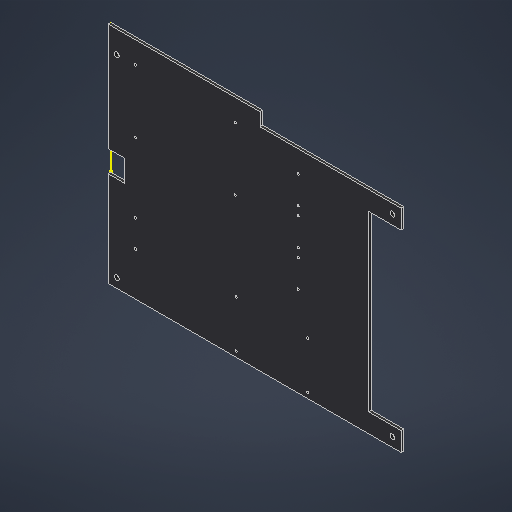
# Autodesk Inventor part: Plate-1
Saved by Autodesk Inventor 2026.2 (Build 302298010, 298A)
## iProperties
Created: 2022-04-19
Part Number: Plate-1
Material: Generic
Document SubType Name: Modeling
Designer: pollak
Density: 1 g/cm^3
Appearance: Default
Author: pollak
Autodesk Inventor part; units mm, degrees
ref_plane "YZ Plane" through (0, 0, 0) normal (1, 0, 0) x (0, 1, 0)
ref_plane "XZ Plane" through (0, 0, 0) normal (0, 1, 0) x (-1, 0, 0)
ref_plane "XY Plane" through (0, 0, 0) normal (0, 0, 1) x (1, 0, 0)
sketch "Sketch1" plane through (0, 0, 0) normal (0, 1, 0) x (-1, 0, 0)
  line L0 (135, 97.5) -> (-135, 97.5)
  line L1 (-135, 97.5) -> (-135, -97.5)
  line L2 (-135, -97.5) -> (135, -97.5)
  line L3 (135, -97.5) -> (135, 97.5)
  line L4 (135, 97.5) -> (-135, -97.5) construction
  line L5 (-135, 97.5) -> (135, -97.5) construction
  line L6 (135, 97.5) -> (-5, 97.5)
  line L7 (-5, 97.5) -> (-5, 109.5)
  line L8 (-5, 109.5) -> (135, 109.5)
  line L9 (135, 109.5) -> (135, 97.5)
  point P0 (0, 0)
  dimension "d0" = 270
  dimension "d1" = 195
  dimension "d2" = 140
  dimension "d3" = 12
  dimension "d4" = 0
  dimension "d5" = 0
  constraints: 20 end point, 4 parallel, 2 horizontal, 2 midpoint, 2 perpendicular
  measures "d0" distance of L2.end L1.end
  measures "d1" distance of L1.end L0.end
  measures "d2" distance of L7.end L8.end
  measures "d3" distance of L6.end L7.end
  measures "d4" distance between parallel lines of L3 L9
  measures "d5" distance between parallel lines of L0 L6
extrude "Extrusion1" add sketch "Sketch1" along normal blind 2.5
sketch "Mounting Holes" plane through (0, 2.5, 0) normal (0, 1, 0) x (1, 0, 0)
  line L0 (-127, -88.9) -> (127, -88.9) construction
  line L1 (127, -88.9) -> (127, 88.9) construction
  line L2 (127, 88.9) -> (-127, 88.9) construction
  line L3 (-127, 88.9) -> (-127, -88.9) construction
  line L4 (-127, -88.9) -> (127, 88.9) construction
  line L5 (127, -88.9) -> (-127, 88.9) construction
  point P0 (0, 0)
  dimension "d32" = 254
  dimension "d33" = 177.8
  constraints: 12 end point, 4 coincident, 2 midpoint, 2 parallel, 1 horizontal, 1 perpendicular
  measures "d32" distance of L2.end L1.end
  measures "d33" distance of L1.end L0.end
hole "Hole3" at (-127, 2.5, -88.9) at (127, 2.5, -88.9) at (127, 2.5, 88.9) at (-127, 2.5, 88.9) direction (0, -1, 0) diameter 4.5 end through all
sketch "Cut" plane through (0, 2.5, 0) normal (0, 1, 0) x (1, 0, 0)
  line L0 (135, 80) -> (105, 80)
  line L1 (105, 80) -> (105, -80)
  line L2 (105, -80) -> (135, -80)
  line L3 (135, -80) -> (135, 80)
  line L4 (135, 80) -> (105, -80) construction
  line L5 (105, 80) -> (135, -80) construction
  line L6 (135, -97.5) -> (135, 97.5) projected
  line L7 (135, 97.5) -> (-135, 97.5) projected
  line L8 (-120, 10) -> (-135, 10)
  line L9 (-135, 10) -> (-135, -10)
  line L10 (-135, -10) -> (-120, -10)
  line L11 (-120, -10) -> (-120, 10)
  line L12 (-120, 10) -> (-135, -10) construction
  line L13 (-135, 10) -> (-120, -10) construction
  line L14 (-135, 97.5) -> (-135, -109.5) projected
  line L15 (135, 72.5) -> (135, 52.5)
  point P0 (0, 0)
  point P1 (120, 0)
  point P2 (-127.5, 0)
  dimension "d62" = 30
  dimension "d63" = 160
  dimension "d64" = 0
  dimension "d65" = 97.5
  dimension "d66" = 15
  dimension "d67" = 20
  dimension "d68" = 0
  dimension "d69" = 97.5
  dimension "d72" = 0
  constraints: 26 end point, 4 midpoint, 4 parallel, 2 horizontal, 2 perpendicular
  measures "d62" distance of L2.end L1.end
  measures "d63" distance of L1.end L0.end
  measures "d64" distance between parallel lines of L6 L3
  measures "d65" distance from line of L7 point (120, 0)
  measures "d66" distance of L10.end L9.end
  measures "d67" distance of L9.end L8.end
  measures "d68" distance between parallel lines of L14 L9
  measures "d69" distance from line of L7 point (-127.5, 0)
  measures "d72" distance between parallel lines of L6 L15
extrude "Plate-cutout" cut sketch "Cut" against normal through all
sketch "Sketch8" plane through (0, 2.5, 0) normal (0, 1, 0) x (1, 0, 0)
  line L0 (5, -109.5) -> (-135, -109.5) construction
  line L1 (-110, -109.5) -> (-110, 97.5) construction
  line L2 (135, 97.5) -> (-135, 97.5) construction
  line L3 (-135, 97.5) -> (-135, -109.5) construction
  line L4 (-135, 10) -> (-120, 10) projected
  line L5 (-120, -10) -> (-135, -10) projected
  point P0 (0, 0)
  point P1 (-110, 57.5)
  point P2 (-110, 32.5)
  dimension "d76" = 25
  dimension "d78" = 25
  dimension "d79" = 40
  dimension "d80" = 22.5
  constraints: 4 point on line, 2 end point, 1 vertical
  measures "d76" distance between parallel lines of L3 L1
  measures "d78" distance of point (-110, 32.5) point (-110, 57.5)
  measures "d79" distance from line of point (-110, 57.5) L2
  measures "d80" distance from line of point (-110, 32.5) L4
hole "Hole6" at (-110, 2.5, -57.5) at (-110, 2.5, -32.5) direction (0, -1, 0) diameter 2.459 end through all thread size "M3x0.5" class "6H" standard "ISO Metric profile"
sketch "Sketch9" plane through (0, 2.5, 0) normal (0, 1, 0) x (1, 0, 0)
  line L0 (-117, 12) -> (-82, 12) construction
  line L1 (-82, 12) -> (-82, 6.5) construction
  line L2 (-82, 6.5) -> (-117, 6.5) construction
  line L3 (-117, 6.5) -> (-117, 12) construction
  line L4 (-135, 97.5) -> (-135, -109.5) projected
  line L5 (-135, 97.5) -> (-135, -109.5) projected
  circle A0 centre (-110, 57.5) radius 1.2295 projected
  point P0 (0, 0)
  point P1 (-135, 10)
  point P2 (-135, -10)
  dimension "d89" = 18
  dimension "d131" = 35
  dimension "d132" = 5.5
  dimension "d133" = 6.5
  constraints: 2 other
  measures "d89" distance between parallel lines of L4 L3
  measures "d131" distance of L3.end L0.end
  measures "d132" distance of L0.end L1.end
  measures "d133" distance from line of point (0, 0) L2
sketch "Sketch10" plane through (0, 2.5, 0) normal (0, 1, 0) x (1, 0, 0)
  line L0 (-17, 92.5) -> (49.04, 92.5) construction
  line L1 (49.04, 92.5) -> (49.04, 49.32) construction
  line L2 (49.04, 49.32) -> (-17, 49.32) construction
  line L3 (-17, 49.32) -> (-17, 92.5) construction
  line L4 (-17, 92.5) -> (49.04, 49.32) construction
  line L5 (49.04, 92.5) -> (-17, 49.32) construction
  line L6 (135, 97.5) -> (-135, 97.5) projected
  line L7 (-135, 97.5) -> (-135, -109.5) projected
  point P0 (0, 0)
  point P1 (16.02, 70.91)
  point P2 (-135, 10)
  dimension "d96" = 66.04
  dimension "d97" = 43.18
  dimension "d98" = 5
  dimension "d99" = 118
  constraints: 12 end point, 4 coincident, 2 midpoint, 2 parallel, 1 horizontal, 1 perpendicular
  measures "d96" distance of L1.end L2.end
  measures "d97" distance of L0.end L1.end
  measures "d98" distance between parallel lines of L0 L6
  measures "d99" distance between parallel lines of L3 L7
hole "B200 mini" at (-17, 2.5, -92.5) at (49.04, 2.5, -92.5) at (49.04, 2.5, -49.32) at (-17, 2.5, -49.32) direction (0, -1, 0) diameter 2.013 end through all thread size "M2.5x0.45" class "6H" standard "ISO Metric profile"
sketch "Sketch11" plane through (0, 2.5, 0) normal (0, 1, 0) x (1, 0, 0)
  line L0 (5, -109.5) -> (-135, -109.5) construction
  line L1 (-18, -109.5) -> (-18, 92.386) construction
  line L2 (-135, 97.5) -> (-135, -109.5) construction
  point P0 (0, 0)
  point P1 (-135, -10)
  point P2 (-18, -89.5)
  point P3 (-18, -31.5)
  point P4 (-110, -89.5)
  point P5 (-110, -31.5)
  dimension "d108" = 58
  dimension "d109" = 20
  dimension "d134" = 92
  dimension "d135" = 25
  constraints: 3 point on line, 2 end point, 2 horizontal alignment, 1 perpendicular, 1 vertical alignment
  measures "d108" distance of point (-18, -31.5) point (-18, -89.5)
  measures "d109" distance from line of point (-18, -89.5) L0
  measures "d134" distance of point (-110, -89.5) point (-18, -89.5)
  measures "d135" distance from line of point (-110, -89.5) L2
hole "RPI" at (-18, 2.5, 89.5) at (-18, 2.5, 31.5) at (-110, 2.5, 89.5) at (-110, 2.5, 31.5) direction (0, -1, 0) diameter 2.013 end through all thread size "M2.5x0.45" class "6H" standard "ISO Metric profile"
sketch "Sketch12" plane through (0, 2.5, 0) normal (0, 1, 0) x (1, 0, 0)
  line L0 (5, -97.5) -> (135, -97.5) projected
  line L1 (40, -97.5) -> (40, 97.2016) construction
  line L2 (-135, 97.5) -> (-135, -109.5) construction
  point P0 (0, 0)
  point P1 (40, 14.7)
  point P2 (40, -10.7)
  point P3 (40, -18.7)
  point P4 (40, -44.1)
  point P5 (40, -52.1)
  point P6 (40, -77.5)
  point P7 (-135, -10)
  dimension "d117" = 25.4
  dimension "d118" = 175
  dimension "d119" = 8
  dimension "d120" = 25.4
  dimension "d121" = 8
  dimension "d122" = 25.4
  dimension "d123" = 20
  constraints: 7 point on line, 2 end point, 1 vertical
  measures "d117" distance of point (40, -10.7) point (40, 14.7)
  measures "d118" distance between parallel lines of L2 L1
  measures "d119" distance of point (40, -10.7) point (40, -18.7)
  measures "d120" distance of point (40, -18.7) point (40, -44.1)
  measures "d121" distance of point (40, -44.1) point (40, -52.1)
  measures "d122" distance of point (40, -52.1) point (40, -77.5)
  measures "d123" distance from line of point (40, -77.5) L0
hole "Mini Circuits" at (40, 2.5, -14.7) at (40, 2.5, 10.7) at (40, 2.5, 18.7) at (40, 2.5, 44.1) at (40, 2.5, 52.1) at (40, 2.5, 77.5) direction (0, -1, 0) diameter 2.013 end through all thread size "M2.5x0.45" class "6H" standard "ISO Metric profile"
body "Solid1"
